Autodesk Fusion 360 part; units mm, degrees
(part 2 of 3)
sketch "Sketch2" plane through (0, 0, 0) normal (0, 0, -1) x (1, 0, 0)
  arc A0 (169.2125, 22.075) -> (169.7125, 21.575) centre (169.7125, 22.075) ccw
  line L0 (169.2125, 22.075) -> (169.2125, 35.075)
  arc A1 (169.7125, 35.575) -> (169.2125, 35.075) centre (169.7125, 35.075) ccw
  line L1 (169.7125, 35.575) -> (182.7125, 35.575)
  arc A2 (183.2125, 35.075) -> (182.7125, 35.575) centre (182.7125, 35.075) ccw
  line L2 (183.2125, 35.075) -> (183.2125, 22.075)
  arc A3 (182.7125, 21.575) -> (183.2125, 22.075) centre (182.7125, 22.075) ccw
  line L3 (182.7125, 21.575) -> (169.7125, 21.575)
  arc A4 (245.4125, 22.075) -> (245.9125, 21.575) centre (245.9125, 22.075) ccw
  line L4 (245.4125, 22.075) -> (245.4125, 35.075)
  arc A5 (245.9125, 35.575) -> (245.4125, 35.075) centre (245.9125, 35.075) ccw
  line L5 (245.9125, 35.575) -> (258.9125, 35.575)
  arc A6 (259.4125, 35.075) -> (258.9125, 35.575) centre (258.9125, 35.075) ccw
  line L6 (259.4125, 35.075) -> (259.4125, 22.075)
  arc A7 (258.9125, 21.575) -> (259.4125, 22.075) centre (258.9125, 22.075) ccw
  line L7 (258.9125, 21.575) -> (245.9125, 21.575)
  arc A8 (354.1625, 2.525) -> (354.6625, 3.025) centre (354.1625, 3.025) ccw
  line L8 (354.1625, 2.525) -> (341.1625, 2.525)
  arc A9 (340.6625, 3.025) -> (341.1625, 2.525) centre (341.1625, 3.025) ccw
  line L9 (340.6625, 3.025) -> (340.6625, 16.025)
  arc A10 (341.1625, 16.525) -> (340.6625, 16.025) centre (341.1625, 16.025) ccw
  line L10 (341.1625, 16.525) -> (354.1625, 16.525)
  arc A11 (354.6625, 16.025) -> (354.1625, 16.525) centre (354.1625, 16.025) ccw
  line L11 (354.6625, 16.025) -> (354.6625, 3.025)
  arc A12 (112.0625, 22.075) -> (112.5625, 21.575) centre (112.5625, 22.075) ccw
  line L12 (112.0625, 22.075) -> (112.0625, 35.075)
  arc A13 (112.5625, 35.575) -> (112.0625, 35.075) centre (112.5625, 35.075) ccw
  line L13 (112.5625, 35.575) -> (125.5625, 35.575)
  arc A14 (126.0625, 35.075) -> (125.5625, 35.575) centre (125.5625, 35.075) ccw
  line L14 (126.0625, 35.075) -> (126.0625, 22.075)
  arc A15 (125.5625, 21.575) -> (126.0625, 22.075) centre (125.5625, 22.075) ccw
  line L15 (125.5625, 21.575) -> (112.5625, 21.575)
  arc A16 (73.9625, 22.075) -> (74.4625, 21.575) centre (74.4625, 22.075) ccw
  line L16 (73.9625, 22.075) -> (73.9625, 35.075)
  arc A17 (74.4625, 35.575) -> (73.9625, 35.075) centre (74.4625, 35.075) ccw
  line L17 (74.4625, 35.575) -> (87.4625, 35.575)
  arc A18 (87.9625, 35.075) -> (87.4625, 35.575) centre (87.4625, 35.075) ccw
  line L18 (87.9625, 35.075) -> (87.9625, 22.075)
  arc A19 (87.4625, 21.575) -> (87.9625, 22.075) centre (87.4625, 22.075) ccw
  line L19 (87.4625, 21.575) -> (74.4625, 21.575)
  arc A20 (283.5125, 22.075) -> (284.0125, 21.575) centre (284.0125, 22.075) ccw
  line L20 (283.5125, 22.075) -> (283.5125, 35.075)
  arc A21 (284.0125, 35.575) -> (283.5125, 35.075) centre (284.0125, 35.075) ccw
  line L21 (284.0125, 35.575) -> (297.0125, 35.575)
  arc A22 (297.5125, 35.075) -> (297.0125, 35.575) centre (297.0125, 35.075) ccw
  line L22 (297.5125, 35.075) -> (297.5125, 22.075)
  arc A23 (297.0125, 21.575) -> (297.5125, 22.075) centre (297.0125, 22.075) ccw
  line L23 (297.0125, 21.575) -> (284.0125, 21.575)
  arc A24 (188.2625, 22.075) -> (188.7625, 21.575) centre (188.7625, 22.075) ccw
  line L24 (188.2625, 22.075) -> (188.2625, 35.075)
  arc A25 (188.7625, 35.575) -> (188.2625, 35.075) centre (188.7625, 35.075) ccw
  line L25 (188.7625, 35.575) -> (201.7625, 35.575)
  arc A26 (202.2625, 35.075) -> (201.7625, 35.575) centre (201.7625, 35.075) ccw
  line L26 (202.2625, 35.075) -> (202.2625, 22.075)
  arc A27 (201.7625, 21.575) -> (202.2625, 22.075) centre (201.7625, 22.075) ccw
  line L27 (201.7625, 21.575) -> (188.7625, 21.575)
  arc A28 (50.15, 22.075) -> (50.65, 21.575) centre (50.65, 22.075) ccw
  line L28 (50.15, 22.075) -> (50.15, 35.075)
  arc A29 (50.65, 35.575) -> (50.15, 35.075) centre (50.65, 35.075) ccw
  line L29 (50.65, 35.575) -> (63.65, 35.575)
  arc A30 (64.15, 35.075) -> (63.65, 35.575) centre (63.65, 35.075) ccw
  line L30 (64.15, 35.075) -> (64.15, 22.075)
  arc A31 (63.65, 21.575) -> (64.15, 22.075) centre (63.65, 22.075) ccw
  line L31 (63.65, 21.575) -> (50.65, 21.575)
  arc A32 (93.0125, 22.075) -> (93.5125, 21.575) centre (93.5125, 22.075) ccw
  line L32 (93.0125, 22.075) -> (93.0125, 35.075)
  arc A33 (93.5125, 35.575) -> (93.0125, 35.075) centre (93.5125, 35.075) ccw
  line L33 (93.5125, 35.575) -> (106.5125, 35.575)
  arc A34 (107.0125, 35.075) -> (106.5125, 35.575) centre (106.5125, 35.075) ccw
  line L34 (107.0125, 35.075) -> (107.0125, 22.075)
  arc A35 (106.5125, 21.575) -> (107.0125, 22.075) centre (106.5125, 22.075) ccw
  line L35 (106.5125, 21.575) -> (93.5125, 21.575)
  arc A36 (359.7125, 3.025) -> (360.2125, 2.525) centre (360.2125, 3.025) ccw
  line L36 (359.7125, 3.025) -> (359.7125, 16.025)
  arc A37 (360.2125, 16.525) -> (359.7125, 16.025) centre (360.2125, 16.025) ccw
  line L37 (360.2125, 16.525) -> (373.2125, 16.525)
  arc A38 (373.7125, 16.025) -> (373.2125, 16.525) centre (373.2125, 16.025) ccw
  line L38 (373.7125, 16.025) -> (373.7125, 3.025)
  arc A39 (373.2125, 2.525) -> (373.7125, 3.025) centre (373.2125, 3.025) ccw
  line L39 (373.2125, 2.525) -> (360.2125, 2.525)
  line L40 (131.1125, 22.075) -> (131.1125, 35.075)
  arc A40 (131.6125, 35.575) -> (131.1125, 35.075) centre (131.6125, 35.075) ccw
  line L41 (131.6125, 35.575) -> (144.6125, 35.575)
  arc A41 (145.1125, 35.075) -> (144.6125, 35.575) centre (144.6125, 35.075) ccw
  line L42 (145.1125, 35.075) -> (145.1125, 22.075)
  arc A42 (144.6125, 21.575) -> (145.1125, 22.075) centre (144.6125, 22.075) ccw
  line L43 (144.6125, 21.575) -> (131.6125, 21.575)
  arc A43 (131.1125, 22.075) -> (131.6125, 21.575) centre (131.6125, 22.075) ccw
  arc A44 (235.8875, 3.025) -> (236.3875, 2.525) centre (236.3875, 3.025) ccw
  line L44 (235.8875, 3.025) -> (235.8875, 16.025)
  arc A45 (236.3875, 16.525) -> (235.8875, 16.025) centre (236.3875, 16.025) ccw
  line L45 (236.3875, 16.525) -> (249.3875, 16.525)
  arc A46 (249.8875, 16.025) -> (249.3875, 16.525) centre (249.3875, 16.025) ccw
  line L46 (249.8875, 16.025) -> (249.8875, 3.025)
  arc A47 (249.3875, 2.525) -> (249.8875, 3.025) centre (249.3875, 3.025) ccw
  line L47 (249.3875, 2.525) -> (236.3875, 2.525)
  line L48 (207.3125, 22.075) -> (207.3125, 35.075)
  arc A48 (207.8125, 35.575) -> (207.3125, 35.075) centre (207.8125, 35.075) ccw
  line L49 (207.8125, 35.575) -> (220.8125, 35.575)
  arc A49 (221.3125, 35.075) -> (220.8125, 35.575) centre (220.8125, 35.075) ccw
  line L50 (221.3125, 35.075) -> (221.3125, 22.075)
  arc A50 (220.8125, 21.575) -> (221.3125, 22.075) centre (220.8125, 22.075) ccw
  line L51 (220.8125, 21.575) -> (207.8125, 21.575)
  arc A51 (207.3125, 22.075) -> (207.8125, 21.575) centre (207.8125, 22.075) ccw
  arc A52 (264.4625, 22.075) -> (264.9625, 21.575) centre (264.9625, 22.075) ccw
  line L52 (264.4625, 22.075) -> (264.4625, 35.075)
  arc A53 (264.9625, 35.575) -> (264.4625, 35.075) centre (264.9625, 35.075) ccw
  line L53 (264.9625, 35.575) -> (277.9625, 35.575)
  arc A54 (278.4625, 35.075) -> (277.9625, 35.575) centre (277.9625, 35.075) ccw
  line L54 (278.4625, 35.075) -> (278.4625, 22.075)
  arc A55 (277.9625, 21.575) -> (278.4625, 22.075) centre (277.9625, 22.075) ccw
  line L55 (277.9625, 21.575) -> (264.9625, 21.575)
  arc A56 (97.775, 41.125) -> (98.275, 40.625) centre (98.275, 41.125) ccw
  line L56 (97.775, 41.125) -> (97.775, 54.125)
  arc A57 (98.275, 54.625) -> (97.775, 54.125) centre (98.275, 54.125) ccw
  line L57 (98.275, 54.625) -> (111.275, 54.625)
  arc A58 (111.775, 54.125) -> (111.275, 54.625) centre (111.275, 54.125) ccw
  line L58 (111.775, 54.125) -> (111.775, 41.125)
  arc A59 (111.275, 40.625) -> (111.775, 41.125) centre (111.275, 41.125) ccw
  line L59 (111.275, 40.625) -> (98.275, 40.625)
  arc A60 (239.8625, 21.575) -> (240.3625, 22.075) centre (239.8625, 22.075) ccw
  line L60 (239.8625, 21.575) -> (226.8625, 21.575)
  arc A61 (226.3625, 22.075) -> (226.8625, 21.575) centre (226.8625, 22.075) ccw
  line L61 (226.3625, 22.075) -> (226.3625, 35.075)
  arc A62 (226.8625, 35.575) -> (226.3625, 35.075) centre (226.8625, 35.075) ccw
  line L62 (226.8625, 35.575) -> (239.8625, 35.575)
  arc A63 (240.3625, 35.075) -> (239.8625, 35.575) centre (239.8625, 35.075) ccw
  line L63 (240.3625, 35.075) -> (240.3625, 22.075)
  arc A64 (307.325, 22.075) -> (307.825, 21.575) centre (307.825, 22.075) ccw
  line L64 (307.325, 22.075) -> (307.325, 35.075)
  arc A65 (307.825, 35.575) -> (307.325, 35.075) centre (307.825, 35.075) ccw
  line L65 (307.825, 35.575) -> (320.825, 35.575)
  arc A66 (321.325, 35.075) -> (320.825, 35.575) centre (320.825, 35.075) ccw
  line L66 (321.325, 35.075) -> (321.325, 22.075)
  arc A67 (320.825, 21.575) -> (321.325, 22.075) centre (320.825, 22.075) ccw
  line L67 (320.825, 21.575) -> (307.825, 21.575)
  arc A68 (116.825, 41.125) -> (117.325, 40.625) centre (117.325, 41.125) ccw
  line L68 (116.825, 41.125) -> (116.825, 54.125)
  arc A69 (117.325, 54.625) -> (116.825, 54.125) centre (117.325, 54.125) ccw
  line L69 (117.325, 54.625) -> (130.325, 54.625)
  arc A70 (130.825, 54.125) -> (130.325, 54.625) centre (130.325, 54.125) ccw
  line L70 (130.825, 54.125) -> (130.825, 41.125)
  arc A71 (130.325, 40.625) -> (130.825, 41.125) centre (130.325, 41.125) ccw
  line L71 (130.325, 40.625) -> (117.325, 40.625)
  arc A72 (354.1625, 21.575) -> (354.6625, 22.075) centre (354.1625, 22.075) ccw
  line L72 (354.1625, 21.575) -> (341.1625, 21.575)
  arc A73 (340.6625, 22.075) -> (341.1625, 21.575) centre (341.1625, 22.075) ccw
  line L73 (340.6625, 22.075) -> (340.6625, 35.075)
  arc A74 (341.1625, 35.575) -> (340.6625, 35.075) centre (341.1625, 35.075) ccw
  line L74 (341.1625, 35.575) -> (354.1625, 35.575)
  arc A75 (354.6625, 35.075) -> (354.1625, 35.575) centre (354.1625, 35.075) ccw
  line L75 (354.6625, 35.075) -> (354.6625, 22.075)
  arc A76 (359.7125, 22.075) -> (360.2125, 21.575) centre (360.2125, 22.075) ccw
  line L76 (359.7125, 22.075) -> (359.7125, 35.075)
  arc A77 (360.2125, 35.575) -> (359.7125, 35.075) centre (360.2125, 35.075) ccw
  line L77 (360.2125, 35.575) -> (373.2125, 35.575)
  arc A78 (373.7125, 35.075) -> (373.2125, 35.575) centre (373.2125, 35.075) ccw
  line L78 (373.7125, 35.075) -> (373.7125, 22.075)
  arc A79 (373.2125, 21.575) -> (373.7125, 22.075) centre (373.2125, 22.075) ccw
  line L79 (373.2125, 21.575) -> (360.2125, 21.575)
  arc A80 (163.6625, 21.575) -> (164.1625, 22.075) centre (163.6625, 22.075) ccw
  line L80 (163.6625, 21.575) -> (150.6625, 21.575)
  arc A81 (150.1625, 22.075) -> (150.6625, 21.575) centre (150.6625, 22.075) ccw
  line L81 (150.1625, 22.075) -> (150.1625, 35.075)
  arc A82 (150.6625, 35.575) -> (150.1625, 35.075) centre (150.6625, 35.075) ccw
  line L82 (150.6625, 35.575) -> (163.6625, 35.575)
  arc A83 (164.1625, 35.075) -> (163.6625, 35.575) centre (163.6625, 35.075) ccw
  line L83 (164.1625, 35.075) -> (164.1625, 22.075)
  arc A84 (92.225, 40.625) -> (92.725, 41.125) centre (92.225, 41.125) ccw
  line L84 (92.225, 40.625) -> (79.225, 40.625)
  arc A85 (78.725, 41.125) -> (79.225, 40.625) centre (79.225, 41.125) ccw
  line L85 (78.725, 41.125) -> (78.725, 54.125)
  arc A86 (79.225, 54.625) -> (78.725, 54.125) centre (79.225, 54.125) ccw
  line L86 (79.225, 54.625) -> (92.225, 54.625)
  arc A87 (92.725, 54.125) -> (92.225, 54.625) centre (92.225, 54.125) ccw
  line L87 (92.725, 54.125) -> (92.725, 41.125)
  line L88 (45.3875, 41.125) -> (45.3875, 54.125)
  arc A88 (45.8875, 54.625) -> (45.3875, 54.125) centre (45.8875, 54.125) ccw
  line L89 (45.8875, 54.625) -> (66.0312, 54.625)
  arc A89 (66.5312, 54.125) -> (66.0312, 54.625) centre (66.0312, 54.125) ccw
  line L90 (66.5312, 54.125) -> (66.5312, 41.125)
  arc A90 (66.0312, 40.625) -> (66.5312, 41.125) centre (66.0312, 41.125) ccw
  line L91 (66.0312, 40.625) -> (45.8875, 40.625)
  arc A91 (45.3875, 41.125) -> (45.8875, 40.625) centre (45.8875, 41.125) ccw
  arc A92 (121.5875, 3.025) -> (122.0875, 2.525) centre (122.0875, 3.025) ccw
  line L92 (121.5875, 3.025) -> (121.5875, 16.025)
  arc A93 (122.0875, 16.525) -> (121.5875, 16.025) centre (122.0875, 16.025) ccw
  line L93 (122.0875, 16.525) -> (135.0875, 16.525)
  arc A94 (135.5875, 16.025) -> (135.0875, 16.525) centre (135.0875, 16.025) ccw
  line L94 (135.5875, 16.025) -> (135.5875, 3.025)
  arc A95 (135.0875, 2.525) -> (135.5875, 3.025) centre (135.0875, 3.025) ccw
  line L95 (135.0875, 2.525) -> (122.0875, 2.525)
  arc A96 (250.175, 41.125) -> (250.675, 40.625) centre (250.675, 41.125) ccw
  line L96 (250.175, 41.125) -> (250.175, 54.125)
  arc A97 (250.675, 54.625) -> (250.175, 54.125) centre (250.675, 54.125) ccw
  line L97 (250.675, 54.625) -> (263.675, 54.625)
  arc A98 (264.175, 54.125) -> (263.675, 54.625) centre (263.675, 54.125) ccw
  line L98 (264.175, 54.125) -> (264.175, 41.125)
  arc A99 (263.675, 40.625) -> (264.175, 41.125) centre (263.675, 41.125) ccw
  line L99 (263.675, 40.625) -> (250.675, 40.625)
  arc A100 (187.475, 40.625) -> (187.975, 41.125) centre (187.475, 41.125) ccw
  line L100 (187.475, 40.625) -> (174.475, 40.625)
  arc A101 (173.975, 41.125) -> (174.475, 40.625) centre (174.475, 41.125) ccw
  line L101 (173.975, 41.125) -> (173.975, 54.125)
  arc A102 (174.475, 54.625) -> (173.975, 54.125) centre (174.475, 54.125) ccw
  line L102 (174.475, 54.625) -> (187.475, 54.625)
  arc A103 (187.975, 54.125) -> (187.475, 54.625) centre (187.475, 54.125) ccw
  line L103 (187.975, 54.125) -> (187.975, 41.125)
  arc A104 (154.925, 41.125) -> (155.425, 40.625) centre (155.425, 41.125) ccw
  line L104 (154.925, 41.125) -> (154.925, 54.125)
  arc A105 (155.425, 54.625) -> (154.925, 54.125) centre (155.425, 54.125) ccw
  line L105 (155.425, 54.625) -> (168.425, 54.625)
  arc A106 (168.925, 54.125) -> (168.425, 54.625) centre (168.425, 54.125) ccw
  line L106 (168.925, 54.125) -> (168.925, 41.125)
  arc A107 (168.425, 40.625) -> (168.925, 41.125) centre (168.425, 41.125) ccw
  line L107 (168.425, 40.625) -> (155.425, 40.625)
  arc A108 (315.6193, 42.125) -> (316.1193, 41.625) centre (316.1193, 42.125) ccw
  line L108 (315.6193, 42.125) -> (315.6193, 56.125)
  arc A109 (316.1193, 56.625) -> (315.6193, 56.125) centre (316.1193, 56.125) ccw
  line L109 (316.1193, 56.625) -> (322.1193, 56.625)
  arc A110 (322.6192, 56.125) -> (322.1193, 56.625) centre (322.1193, 56.125) ccw
  line L110 (322.6192, 56.125) -> (322.6192, 42.125)
  arc A111 (322.1193, 41.625) -> (322.6192, 42.125) centre (322.1193, 42.125) ccw
  line L111 (322.1193, 41.625) -> (316.1193, 41.625)
  arc A112 (72.7318, 61.175) -> (73.2318, 60.675) centre (73.2318, 61.175) ccw
  line L112 (72.7318, 61.175) -> (72.7318, 75.175)
  arc A113 (73.2318, 75.675) -> (72.7318, 75.175) centre (73.2318, 75.175) ccw
  line L113 (73.2318, 75.675) -> (79.2318, 75.675)
  arc A114 (79.7318, 75.175) -> (79.2318, 75.675) centre (79.2318, 75.175) ccw
  line L114 (79.7318, 75.175) -> (79.7318, 61.175)
  arc A115 (79.2318, 60.675) -> (79.7318, 61.175) centre (79.2318, 61.175) ccw
  line L115 (79.2318, 60.675) -> (73.2318, 60.675)
  arc A116 (139.85, 59.675) -> (140.35, 60.175) centre (139.85, 60.175) ccw
  line L116 (139.85, 59.675) -> (126.85, 59.675)
  arc A117 (126.35, 60.175) -> (126.85, 59.675) centre (126.85, 60.175) ccw
  line L117 (126.35, 60.175) -> (126.35, 73.175)
  arc A118 (126.85, 73.675) -> (126.35, 73.175) centre (126.85, 73.175) ccw
  line L118 (126.85, 73.675) -> (139.85, 73.675)
  arc A119 (140.35, 73.175) -> (139.85, 73.675) centre (139.85, 73.175) ccw
  line L119 (140.35, 73.175) -> (140.35, 60.175)
  line L120 (145.4, 60.175) -> (145.4, 73.175)
  arc A120 (145.9, 73.675) -> (145.4, 73.175) centre (145.9, 73.175) ccw
  line L121 (145.9, 73.675) -> (158.9, 73.675)
  arc A121 (159.4, 73.175) -> (158.9, 73.675) centre (158.9, 73.175) ccw
  line L122 (159.4, 73.175) -> (159.4, 60.175)
  arc A122 (158.9, 59.675) -> (159.4, 60.175) centre (158.9, 60.175) ccw
  line L123 (158.9, 59.675) -> (145.9, 59.675)
  arc A123 (145.4, 60.175) -> (145.9, 59.675) centre (145.9, 60.175) ccw
  arc A124 (183.5, 60.175) -> (184, 59.675) centre (184, 60.175) ccw
  line L124 (183.5, 60.175) -> (183.5, 73.175)
  arc A125 (184, 73.675) -> (183.5, 73.175) centre (184, 73.175) ccw
  line L125 (184, 73.675) -> (197, 73.675)
  arc A126 (197.5, 73.175) -> (197, 73.675) centre (197, 73.175) ccw
  line L126 (197.5, 73.175) -> (197.5, 60.175)
  arc A127 (197, 59.675) -> (197.5, 60.175) centre (197, 60.175) ccw
  line L127 (197, 59.675) -> (184, 59.675)
  arc A128 (48.8558, 61.175) -> (49.3558, 60.675) centre (49.3558, 61.175) ccw
  line L128 (48.8558, 61.175) -> (48.8558, 75.175)
  arc A129 (49.3558, 75.675) -> (48.8558, 75.175) centre (49.3558, 75.175) ccw
  line L129 (49.3558, 75.675) -> (55.3558, 75.675)
  arc A130 (55.8558, 75.175) -> (55.3558, 75.675) centre (55.3558, 75.175) ccw
  line L130 (55.8558, 75.175) -> (55.8558, 61.175)
  arc A131 (55.3558, 60.675) -> (55.8558, 61.175) centre (55.3558, 61.175) ccw
  line L131 (55.3558, 60.675) -> (49.3558, 60.675)
  arc A132 (340.6625, 60.175) -> (341.1625, 59.675) centre (341.1625, 60.175) ccw
  line L132 (340.6625, 60.175) -> (340.6625, 73.175)
  arc A133 (341.1625, 73.675) -> (340.6625, 73.175) centre (341.1625, 73.175) ccw
  line L133 (341.1625, 73.675) -> (354.1625, 73.675)
  arc A134 (354.6625, 73.175) -> (354.1625, 73.675) centre (354.1625, 73.175) ccw
  line L134 (354.6625, 73.175) -> (354.6625, 60.175)
  arc A135 (354.1625, 59.675) -> (354.6625, 60.175) centre (354.1625, 60.175) ccw
  line L135 (354.1625, 59.675) -> (341.1625, 59.675)
  arc A136 (164.45, 60.175) -> (164.95, 59.675) centre (164.95, 60.175) ccw
  line L136 (164.45, 60.175) -> (164.45, 73.175)
  arc A137 (164.95, 73.675) -> (164.45, 73.175) centre (164.95, 73.175) ccw
  line L137 (164.95, 73.675) -> (177.95, 73.675)
  arc A138 (178.45, 73.175) -> (177.95, 73.675) centre (177.95, 73.175) ccw
  line L138 (178.45, 73.175) -> (178.45, 60.175)
  arc A139 (177.95, 59.675) -> (178.45, 60.175) centre (177.95, 60.175) ccw
  line L139 (177.95, 59.675) -> (164.95, 59.675)
  arc A140 (259.7, 60.175) -> (260.2, 59.675) centre (260.2, 60.175) ccw
  line L140 (259.7, 60.175) -> (259.7, 73.175)
  arc A141 (260.2, 73.675) -> (259.7, 73.175) centre (260.2, 73.175) ccw
  line L141 (260.2, 73.675) -> (273.2, 73.675)
  arc A142 (273.7, 73.175) -> (273.2, 73.675) centre (273.2, 73.175) ccw
  line L142 (273.7, 73.175) -> (273.7, 60.175)
  arc A143 (273.2, 59.675) -> (273.7, 60.175) centre (273.2, 60.175) ccw
  line L143 (273.2, 59.675) -> (260.2, 59.675)
  arc A144 (313.6812, 40.625) -> (314.1812, 41.125) centre (313.6812, 41.125) ccw
  line L144 (313.6812, 40.625) -> (300.6812, 40.625)
  arc A145 (300.1812, 41.125) -> (300.6812, 40.625) centre (300.6812, 41.125) ccw
  line L145 (300.1812, 41.125) -> (300.1812, 54.125)
  arc A146 (300.6812, 54.625) -> (300.1812, 54.125) centre (300.6812, 54.125) ccw
  line L146 (300.6812, 54.625) -> (313.6812, 54.625)
  arc A147 (314.1812, 54.125) -> (313.6812, 54.625) centre (313.6812, 54.125) ccw
  line L147 (314.1812, 54.125) -> (314.1812, 41.125)
  arc A148 (135.875, 41.125) -> (136.375, 40.625) centre (136.375, 41.125) ccw
  line L148 (135.875, 41.125) -> (135.875, 54.125)
  arc A149 (136.375, 54.625) -> (135.875, 54.125) centre (136.375, 54.125) ccw
  line L149 (136.375, 54.625) -> (149.375, 54.625)
  arc A150 (149.875, 54.125) -> (149.375, 54.625) centre (149.375, 54.125) ccw
  line L150 (149.875, 54.125) -> (149.875, 41.125)
  arc A151 (149.375, 40.625) -> (149.875, 41.125) centre (149.375, 41.125) ccw
  line L151 (149.375, 40.625) -> (136.375, 40.625)
  arc A152 (166.8313, 79.225) -> (167.3313, 78.725) centre (167.3313, 79.225) ccw
  line L152 (166.8313, 79.225) -> (166.8313, 92.225)
  arc A153 (167.3313, 92.725) -> (166.8313, 92.225) centre (167.3313, 92.225) ccw
  line L153 (167.3313, 92.725) -> (180.3313, 92.725)
  arc A154 (180.8313, 92.225) -> (180.3313, 92.725) centre (180.3313, 92.225) ccw
  line L154 (180.8313, 92.225) -> (180.8313, 79.225)
  arc A155 (180.3313, 78.725) -> (180.8313, 79.225) centre (180.3313, 79.225) ccw
  line L155 (180.3313, 78.725) -> (167.3313, 78.725)
  line L156 (107.3, 60.175) -> (107.3, 73.175)
  arc A156 (107.8, 73.675) -> (107.3, 73.175) centre (107.8, 73.175) ccw
  line L157 (107.8, 73.675) -> (120.8, 73.675)
  arc A157 (121.3, 73.175) -> (120.8, 73.675) centre (120.8, 73.175) ccw
  line L158 (121.3, 73.175) -> (121.3, 60.175)
  arc A158 (120.8, 59.675) -> (121.3, 60.175) centre (120.8, 60.175) ccw
  line L159 (120.8, 59.675) -> (107.8, 59.675)
  arc A159 (107.3, 60.175) -> (107.8, 59.675) centre (107.8, 60.175) ccw
  arc A160 (291.7432, 42.125) -> (292.2432, 41.625) centre (292.2432, 42.125) ccw
  line L160 (291.7432, 42.125) -> (291.7432, 56.125)
  arc A161 (292.2432, 56.625) -> (291.7432, 56.125) centre (292.2432, 56.125) ccw
  line L161 (292.2432, 56.625) -> (298.2432, 56.625)
  arc A162 (298.7432, 56.125) -> (298.2432, 56.625) centre (298.2432, 56.125) ccw
  line L162 (298.7433, 56.125) -> (298.7433, 42.125)
  arc A163 (298.2432, 41.625) -> (298.7432, 42.125) centre (298.2432, 42.125) ccw
  line L163 (298.2432, 41.625) -> (292.2432, 41.625)
  arc A164 (220.3313, 80.225) -> (220.8313, 79.725) centre (220.8313, 80.225) ccw
  line L164 (220.3313, 80.225) -> (220.3313, 94.225)
  arc A165 (220.8313, 94.725) -> (220.3313, 94.225) centre (220.8313, 94.225) ccw
  line L165 (220.8313, 94.725) -> (226.8313, 94.725)
  arc A166 (227.3313, 94.225) -> (226.8313, 94.725) centre (226.8313, 94.225) ccw
  line L166 (227.3313, 94.225) -> (227.3313, 80.225)
  arc A167 (226.8313, 79.725) -> (227.3313, 80.225) centre (226.8313, 80.225) ccw
  line L167 (226.8313, 79.725) -> (220.8313, 79.725)
  arc A168 (120.3313, 80.225) -> (120.8313, 79.725) centre (120.8313, 80.225) ccw
  line L168 (120.3313, 80.225) -> (120.3312, 94.225)
  arc A169 (120.8313, 94.725) -> (120.3313, 94.225) centre (120.8313, 94.225) ccw
  line L169 (120.8313, 94.725) -> (126.8313, 94.725)
  arc A170 (127.3313, 94.225) -> (126.8313, 94.725) centre (126.8313, 94.225) ccw
  line L170 (127.3313, 94.225) -> (127.3313, 80.225)
  arc A171 (126.8313, 79.725) -> (127.3313, 80.225) centre (126.8313, 80.225) ccw
  line L171 (126.8313, 79.725) -> (120.8313, 79.725)
  arc A172 (95.3938, 79.225) -> (95.8938, 78.725) centre (95.8938, 79.225) ccw
  line L172 (95.3937, 79.225) -> (95.3937, 92.225)
  arc A173 (95.8938, 92.725) -> (95.3938, 92.225) centre (95.8938, 92.225) ccw
  line L173 (95.8938, 92.725) -> (108.8938, 92.725)
  arc A174 (109.3938, 92.225) -> (108.8938, 92.725) centre (108.8938, 92.225) ccw
  line L174 (109.3938, 92.225) -> (109.3938, 79.225)
  arc A175 (108.8938, 78.725) -> (109.3938, 79.225) centre (108.8938, 79.225) ccw
  line L175 (108.8938, 78.725) -> (95.8938, 78.725)
  arc A176 (202.55, 60.175) -> (203.05, 59.675) centre (203.05, 60.175) ccw
  line L176 (202.55, 60.175) -> (202.55, 73.175)
  arc A177 (203.05, 73.675) -> (202.55, 73.175) centre (203.05, 73.175) ccw
  line L177 (203.05, 73.675) -> (216.05, 73.675)
  arc A178 (216.55, 73.175) -> (216.05, 73.675) centre (216.05, 73.175) ccw
  line L178 (216.55, 73.175) -> (216.55, 60.175)
  arc A179 (216.05, 59.675) -> (216.55, 60.175) centre (216.05, 60.175) ccw
  line L179 (216.05, 59.675) -> (203.05, 59.675)
  arc A180 (88.25, 60.175) -> (88.75, 59.675) centre (88.75, 60.175) ccw
  line L180 (88.25, 60.175) -> (88.25, 73.175)
  arc A181 (88.75, 73.675) -> (88.25, 73.175) centre (88.75, 73.175) ccw
  line L181 (88.75, 73.675) -> (101.75, 73.675)
  arc A182 (102.25, 73.175) -> (101.75, 73.675) centre (101.75, 73.175) ccw
  line L182 (102.25, 73.175) -> (102.25, 60.175)
  arc A183 (101.75, 59.675) -> (102.25, 60.175) centre (101.75, 60.175) ccw
  line L183 (101.75, 59.675) -> (88.75, 59.675)
  line L184 (240.65, 60.175) -> (240.65, 73.175)
  arc A184 (241.15, 73.675) -> (240.65, 73.175) centre (241.15, 73.175) ccw
  line L185 (241.15, 73.675) -> (254.15, 73.675)
  arc A185 (254.65, 73.175) -> (254.15, 73.675) centre (254.15, 73.175) ccw
  line L186 (254.65, 73.175) -> (254.65, 60.175)
  arc A186 (254.15, 59.675) -> (254.65, 60.175) centre (254.15, 60.175) ccw
  line L187 (254.15, 59.675) -> (241.15, 59.675)
  arc A187 (240.65, 60.175) -> (241.15, 59.675) centre (241.15, 60.175) ccw
  arc A188 (221.6, 60.175) -> (222.1, 59.675) centre (222.1, 60.175) ccw
  line L188 (221.6, 60.175) -> (221.6, 73.175)
  arc A189 (222.1, 73.675) -> (221.6, 73.175) centre (222.1, 73.175) ccw
  line L189 (222.1, 73.675) -> (235.1, 73.675)
  arc A190 (235.6, 73.175) -> (235.1, 73.675) centre (235.1, 73.175) ccw
  line L190 (235.6, 73.175) -> (235.6, 60.175)
  arc A191 (235.1, 59.675) -> (235.6, 60.175) centre (235.1, 60.175) ccw
  line L191 (235.1, 59.675) -> (222.1, 59.675)
  arc A192 (262.0813, 79.225) -> (262.5813, 78.725) centre (262.5813, 79.225) ccw
  line L192 (262.0813, 79.225) -> (262.0813, 92.225)
  arc A193 (262.5813, 92.725) -> (262.0813, 92.225) centre (262.5813, 92.225) ccw
  line L193 (262.5813, 92.725) -> (275.5813, 92.725)
  arc A194 (276.0813, 92.225) -> (275.5813, 92.725) centre (275.5813, 92.225) ccw
  line L194 (276.0813, 92.225) -> (276.0813, 79.225)
  arc A195 (275.5813, 78.725) -> (276.0813, 79.225) centre (275.5813, 79.225) ccw
  line L195 (275.5813, 78.725) -> (262.5813, 78.725)
  arc A196 (231.125, 41.125) -> (231.625, 40.625) centre (231.625, 41.125) ccw
  line L196 (231.125, 41.125) -> (231.125, 54.125)
  arc A197 (231.625, 54.625) -> (231.125, 54.125) centre (231.625, 54.125) ccw
  line L197 (231.625, 54.625) -> (244.625, 54.625)
  arc A198 (245.125, 54.125) -> (244.625, 54.625) centre (244.625, 54.125) ccw
  line L198 (245.125, 54.125) -> (245.125, 41.125)
  arc A199 (244.625, 40.625) -> (245.125, 41.125) centre (244.625, 41.125) ccw
  line L199 (244.625, 40.625) -> (231.625, 40.625)
  arc A200 (71.5812, 79.225) -> (72.0812, 78.725) centre (72.0812, 79.225) ccw
  line L200 (71.5812, 79.225) -> (71.5812, 92.225)
  arc A201 (72.0812, 92.725) -> (71.5812, 92.225) centre (72.0812, 92.225) ccw
  line L201 (72.0812, 92.725) -> (85.0812, 92.725)
  arc A202 (85.5813, 92.225) -> (85.0812, 92.725) centre (85.0812, 92.225) ccw
  line L202 (85.5813, 92.225) -> (85.5813, 79.225)
  arc A203 (85.0812, 78.725) -> (85.5813, 79.225) centre (85.0812, 79.225) ccw
  line L203 (85.0812, 78.725) -> (72.0812, 78.725)
  arc A204 (463.5139, 44.7152) -> (463.5139, 48.8568) centre (463.5139, 46.786) ccw
  line L204 (463.5139, 44.7152) -> (459.7929, 44.7152)
  line L205 (459.7929, 44.7152) -> (459.7929, 34.7152)
  line L206 (459.7929, 34.7152) -> (383.7929, 34.7152)
  line L207 (383.7929, 34.7152) -> (383.7929, 44.7152)
  line L208 (383.7929, 44.7152) -> (380.072, 44.7152)
  arc A205 (380.072, 48.8568) -> (380.072, 44.7152) centre (380.072, 46.786) ccw
  line L209 (380.072, 48.8568) -> (383.7929, 48.8568)
  line L210 (383.7929, 48.8568) -> (383.7929, 88.7152)
  line L211 (383.7929, 88.7152) -> (459.7929, 88.7152)
  line L212 (459.7929, 88.7152) -> (459.7929, 48.8568)
  line L213 (459.7929, 48.8568) -> (463.5139, 48.8568)
  arc A206 (287.4808, 75.675) -> (286.9808, 75.175) centre (287.4808, 75.175) ccw
  line L214 (287.4808, 75.675) -> (293.4808, 75.675)
  arc A207 (293.9808, 75.175) -> (293.4808, 75.675) centre (293.4808, 75.175) ccw
  line L215 (293.9808, 75.175) -> (293.9808, 74.175)
  arc A208 (293.9808, 74.175) -> (294.4808, 73.675) centre (294.4807, 74.175) ccw
  line L216 (294.4808, 73.675) -> (308.9188, 73.675)
  arc A209 (309.4187, 73.175) -> (308.9187, 73.675) centre (308.9187, 73.175) ccw
  line L217 (309.4187, 73.175) -> (309.4187, 60.175)
  arc A210 (308.9187, 59.675) -> (309.4187, 60.175) centre (308.9187, 60.175) ccw
  line L218 (308.9187, 59.675) -> (286.3937, 59.675)
  arc A211 (285.8937, 60.175) -> (286.3937, 59.675) centre (286.3937, 60.175) ccw
  line L219 (285.8937, 60.175) -> (285.8938, 73.175)
  arc A212 (286.3937, 73.675) -> (285.8937, 73.175) centre (286.3937, 73.175) ccw
  line L220 (286.3937, 73.675) -> (286.4808, 73.675)
  arc A213 (286.4808, 73.675) -> (286.9808, 74.175) centre (286.4808, 74.175) ccw
  line L221 (286.9808, 74.175) -> (286.9808, 75.175)
  arc A214 (238.2688, 79.225) -> (238.7688, 78.725) centre (238.7688, 79.225) ccw
  line L222 (238.2688, 79.225) -> (238.2688, 92.225)
  arc A215 (238.7688, 92.725) -> (238.2688, 92.225) centre (238.7688, 92.225) ccw
  line L223 (238.7688, 92.725) -> (251.7687, 92.725)
  arc A216 (252.2687, 92.225) -> (251.7687, 92.725) centre (251.7687, 92.225) ccw
  line L224 (252.2688, 92.225) -> (252.2688, 79.225)
  arc A217 (251.7687, 78.725) -> (252.2687, 79.225) centre (251.7687, 79.225) ccw
  line L225 (251.7687, 78.725) -> (238.7688, 78.725)
  line L226 (273.9875, 3.025) -> (273.9875, 16.025)
  arc A218 (274.4875, 16.525) -> (273.9875, 16.025) centre (274.4875, 16.025) ccw
  line L227 (274.4875, 16.525) -> (287.4875, 16.525)
  arc A219 (287.9875, 16.025) -> (287.4875, 16.525) centre (287.4875, 16.025) ccw
  line L228 (287.9875, 16.025) -> (287.9875, 3.025)
  arc A220 (287.4875, 2.525) -> (287.9875, 3.025) centre (287.4875, 3.025) ccw
  line L229 (287.4875, 2.525) -> (274.4875, 2.525)
  arc A221 (273.9875, 3.025) -> (274.4875, 2.525) centre (274.4875, 3.025) ccw
  arc A222 (326.0875, 73.175) -> (325.5875, 73.675) centre (325.5875, 73.175) ccw
  line L230 (326.0875, 73.175) -> (326.0875, 60.175)
  arc A223 (325.5875, 59.675) -> (326.0875, 60.175) centre (325.5875, 60.175) ccw
  line L231 (325.5875, 59.675) -> (312.5875, 59.675)
  arc A224 (312.0875, 60.175) -> (312.5875, 59.675) centre (312.5875, 60.175) ccw
  arc A225 (312.0875, 60.175) -> (311.5875, 60.675) centre (311.5875, 60.175) ccw
  line L232 (311.5875, 60.675) -> (311.3567, 60.675)
  arc A226 (310.8567, 61.175) -> (311.3567, 60.675) centre (311.3567, 61.175) ccw
  line L233 (310.8567, 61.175) -> (310.8567, 75.175)
  arc A227 (311.3567, 75.675) -> (310.8567, 75.175) centre (311.3567, 75.175) ccw
  line L234 (311.3567, 75.675) -> (317.3567, 75.675)
  arc A228 (317.8568, 75.175) -> (317.3568, 75.675) centre (317.3568, 75.175) ccw
  line L235 (317.8568, 75.175) -> (317.8568, 74.175)
  arc A229 (317.8568, 74.175) -> (318.3568, 73.675) centre (318.3567, 74.175) ccw
  line L236 (318.3568, 73.675) -> (325.5875, 73.675)
  arc A230 (254.9375, 3.025) -> (255.4375, 2.525) centre (255.4375, 3.025) ccw
  line L237 (254.9375, 3.025) -> (254.9375, 16.025)
  arc A231 (255.4375, 16.525) -> (254.9375, 16.025) centre (255.4375, 16.025) ccw
  line L238 (255.4375, 16.525) -> (268.4375, 16.525)
  arc A232 (268.9375, 16.025) -> (268.4375, 16.525) centre (268.4375, 16.025) ccw
  line L239 (268.9375, 16.025) -> (268.9375, 3.025)
  arc A233 (268.4375, 2.525) -> (268.9375, 3.025) centre (268.4375, 3.025) ccw
  line L240 (268.4375, 2.525) -> (255.4375, 2.525)
  arc A234 (326.0875, 16.025) -> (325.5875, 16.525) centre (325.5875, 16.025) ccw
  line L241 (326.0875, 16.025) -> (326.0875, 3.025)
  arc A235 (325.5875, 2.525) -> (326.0875, 3.025) centre (325.5875, 3.025) ccw
  line L242 (325.5875, 2.525) -> (293.5375, 2.525)
  arc A236 (293.0375, 3.025) -> (293.5375, 2.525) centre (293.5375, 3.025) ccw
  line L243 (293.0375, 3.025) -> (293.0375, 16.025)
  arc A237 (293.5375, 16.525) -> (293.0375, 16.025) centre (293.5375, 16.025) ccw
  line L244 (293.5375, 16.525) -> (293.6245, 16.525)
  arc A238 (293.6245, 16.525) -> (294.1245, 17.025) centre (293.6245, 17.025) ccw
  line L245 (294.1245, 17.025) -> (294.1245, 18.025)
  arc A239 (294.6245, 18.525) -> (294.1245, 18.025) centre (294.6245, 18.025) ccw
  line L246 (294.6245, 18.525) -> (300.6245, 18.525)
  arc A240 (301.1245, 18.025) -> (300.6245, 18.525) centre (300.6245, 18.025) ccw
  line L247 (301.1245, 18.025) -> (301.1245, 17.025)
  arc A241 (301.1245, 17.025) -> (301.6245, 16.525) centre (301.6245, 17.025) ccw
  line L248 (301.6245, 16.525) -> (317.5005, 16.525)
  arc A242 (317.5005, 16.525) -> (318.0005, 17.025) centre (317.5005, 17.025) ccw
  line L249 (318.0005, 17.025) -> (318.0005, 18.025)
  arc A243 (318.5005, 18.525) -> (318.0005, 18.025) centre (318.5005, 18.025) ccw
  line L250 (318.5005, 18.525) -> (324.5005, 18.525)
  arc A244 (325.0005, 18.025) -> (324.5005, 18.525) centre (324.5005, 18.025) ccw
  line L251 (325.0005, 18.025) -> (325.0005, 17.025)
  arc A245 (325.0005, 17.025) -> (325.5005, 16.525) centre (325.5005, 17.025) ccw
  line L252 (325.5005, 16.525) -> (325.5875, 16.525)
  arc A246 (212.075, 41.125) -> (212.575, 40.625) centre (212.575, 41.125) ccw
  line L253 (212.075, 41.125) -> (212.075, 54.125)
  arc A247 (212.575, 54.625) -> (212.075, 54.125) centre (212.575, 54.125) ccw
  line L254 (212.575, 54.625) -> (225.575, 54.625)
  arc A248 (226.075, 54.125) -> (225.575, 54.625) centre (225.575, 54.125) ccw
  line L255 (226.075, 54.125) -> (226.075, 41.125)
  arc A249 (225.575, 40.625) -> (226.075, 41.125) centre (225.575, 41.125) ccw
  line L256 (225.575, 40.625) -> (212.575, 40.625)
  arc A250 (57.2938, 60.175) -> (57.7938, 59.675) centre (57.7938, 60.175) ccw
  line L257 (57.2938, 60.175) -> (57.2938, 73.175)
  arc A251 (57.7938, 73.675) -> (57.2938, 73.175) centre (57.7938, 73.175) ccw
  line L258 (57.7938, 73.675) -> (70.7938, 73.675)
  arc A252 (71.2938, 73.175) -> (70.7938, 73.675) centre (70.7938, 73.175) ccw
  line L259 (71.2938, 73.175) -> (71.2938, 60.175)
  arc A253 (70.7938, 59.675) -> (71.2938, 60.175) centre (70.7938, 60.175) ccw
  line L260 (70.7938, 59.675) -> (57.7938, 59.675)
  arc A254 (321.6125, 79.225) -> (322.1125, 78.725) centre (322.1125, 79.225) ccw
  line L261 (321.6125, 79.225) -> (321.6125, 92.225)
  arc A255 (322.1125, 92.725) -> (321.6125, 92.225) centre (322.1125, 92.225) ccw
  line L262 (322.1125, 92.725) -> (335.1125, 92.725)
  arc A256 (335.6125, 92.225) -> (335.1125, 92.725) centre (335.1125, 92.225) ccw
  line L263 (335.6125, 92.225) -> (335.6125, 79.225)
  arc A257 (335.1125, 78.725) -> (335.6125, 79.225) centre (335.1125, 79.225) ccw
  line L264 (335.1125, 78.725) -> (322.1125, 78.725)
  arc A258 (193.025, 41.125) -> (193.525, 40.625) centre (193.525, 41.125) ccw
  line L265 (193.025, 41.125) -> (193.025, 54.125)
  arc A259 (193.525, 54.625) -> (193.025, 54.125) centre (193.525, 54.125) ccw
  line L266 (193.525, 54.625) -> (206.525, 54.625)
  arc A260 (207.025, 54.125) -> (206.525, 54.625) centre (206.525, 54.125) ccw
  line L267 (207.025, 54.125) -> (207.025, 41.125)
  arc A261 (206.525, 40.625) -> (207.025, 41.125) centre (206.525, 41.125) ccw
  line L268 (206.525, 40.625) -> (193.525, 40.625)
  arc A262 (285.8938, 79.225) -> (286.3938, 78.725) centre (286.3938, 79.225) ccw
  line L269 (285.8938, 79.225) -> (285.8938, 92.225)
  arc A263 (286.3938, 92.725) -> (285.8938, 92.225) centre (286.3938, 92.225) ccw
  line L270 (286.3938, 92.725) -> (299.3938, 92.725)
  arc A264 (299.8938, 92.225) -> (299.3938, 92.725) centre (299.3938, 92.225) ccw
  line L271 (299.8938, 92.225) -> (299.8938, 79.225)
  arc A265 (299.3938, 78.725) -> (299.8938, 79.225) centre (299.3938, 79.225) ccw
  line L272 (299.3938, 78.725) -> (286.3938, 78.725)
  arc A266 (159.6875, 3.025) -> (160.1875, 2.525) centre (160.1875, 3.025) ccw
  line L273 (159.6875, 3.025) -> (159.6875, 16.025)
  arc A267 (160.1875, 16.525) -> (159.6875, 16.025) centre (160.1875, 16.025) ccw
  line L274 (160.1875, 16.525) -> (173.1875, 16.525)
  arc A268 (173.6875, 16.025) -> (173.1875, 16.525) centre (173.1875, 16.025) ccw
  line L275 (173.6875, 16.025) -> (173.6875, 3.025)
  arc A269 (173.1875, 2.525) -> (173.6875, 3.025) centre (173.1875, 3.025) ccw
  line L276 (173.1875, 2.525) -> (160.1875, 2.525)
  arc A270 (359.7125, 79.225) -> (360.2125, 78.725) centre (360.2125, 79.225) ccw
  line L277 (359.7125, 79.225) -> (359.7125, 92.225)
  arc A271 (360.2125, 92.725) -> (359.7125, 92.225) centre (360.2125, 92.225) ccw
  line L278 (360.2125, 92.725) -> (373.2125, 92.725)
  arc A272 (373.7125, 92.225) -> (373.2125, 92.725) centre (373.2125, 92.225) ccw
  line L279 (373.7125, 92.225) -> (373.7125, 79.225)
  arc A273 (373.2125, 78.725) -> (373.7125, 79.225) centre (373.2125, 79.225) ccw
  line L280 (373.2125, 78.725) -> (360.2125, 78.725)
  arc A274 (282.725, 40.625) -> (283.225, 41.125) centre (282.725, 41.125) ccw
  line L281 (282.725, 40.625) -> (269.725, 40.625)
  arc A275 (269.225, 41.125) -> (269.725, 40.625) centre (269.725, 41.125) ccw
  line L282 (269.225, 41.125) -> (269.225, 54.125)
  arc A276 (269.725, 54.625) -> (269.225, 54.125) centre (269.725, 54.125) ccw
  line L283 (269.725, 54.625) -> (282.725, 54.625)
  arc A277 (283.225, 54.125) -> (282.725, 54.625) centre (282.725, 54.125) ccw
  line L284 (283.225, 54.125) -> (283.225, 41.125)
  arc A278 (83.4875, 3.025) -> (83.9875, 2.525) centre (83.9875, 3.025) ccw
  line L285 (83.4875, 3.025) -> (83.4875, 16.025)
  arc A279 (83.9875, 16.525) -> (83.4875, 16.025) centre (83.9875, 16.025) ccw
  line L286 (83.9875, 16.525) -> (96.9875, 16.525)
  arc A280 (97.4875, 16.025) -> (96.9875, 16.525) centre (96.9875, 16.025) ccw
  line L287 (97.4875, 16.025) -> (97.4875, 3.025)
  arc A281 (96.9875, 2.525) -> (97.4875, 3.025) centre (96.9875, 3.025) ccw
  line L288 (96.9875, 2.525) -> (83.9875, 2.525)
  arc A282 (64.4375, 3.025) -> (64.9375, 2.525) centre (64.9375, 3.025) ccw
  line L289 (64.4375, 3.025) -> (64.4375, 16.025)
  arc A283 (64.9375, 16.525) -> (64.4375, 16.025) centre (64.9375, 16.025) ccw
  line L290 (64.9375, 16.525) -> (77.9375, 16.525)
  arc A284 (78.4375, 16.025) -> (77.9375, 16.525) centre (77.9375, 16.025) ccw
  line L291 (78.4375, 16.025) -> (78.4375, 3.025)
  arc A285 (77.9375, 2.525) -> (78.4375, 3.025) centre (77.9375, 3.025) ccw
  line L292 (77.9375, 2.525) -> (64.9375, 2.525)
  arc A286 (340.6625, 79.225) -> (341.1625, 78.725) centre (341.1625, 79.225) ccw
  line L293 (340.6625, 79.225) -> (340.6625, 92.225)
  arc A287 (341.1625, 92.725) -> (340.6625, 92.225) centre (341.1625, 92.225) ccw
  line L294 (341.1625, 92.725) -> (354.1625, 92.725)
  arc A288 (354.6625, 92.225) -> (354.1625, 92.725) centre (354.1625, 92.225) ccw
  line L295 (354.6625, 92.225) -> (354.6625, 79.225)
  arc A289 (354.1625, 78.725) -> (354.6625, 79.225) centre (354.1625, 79.225) ccw
  line L296 (354.1625, 78.725) -> (341.1625, 78.725)
  arc A290 (140.6375, 3.025) -> (141.1375, 2.525) centre (141.1375, 3.025) ccw
  line L297 (140.6375, 3.025) -> (140.6375, 16.025)
  arc A291 (141.1375, 16.525) -> (140.6375, 16.025) centre (141.1375, 16.025) ccw
  line L298 (141.1375, 16.525) -> (154.1375, 16.525)
  arc A292 (154.6375, 16.025) -> (154.1375, 16.525) centre (154.1375, 16.025) ccw
  line L299 (154.6375, 16.025) -> (154.6375, 3.025)
  arc A293 (154.1375, 2.525) -> (154.6375, 3.025) centre (154.1375, 3.025) ccw
  line L300 (154.1375, 2.525) -> (141.1375, 2.525)
  arc A294 (178.7375, 3.025) -> (179.2375, 2.525) centre (179.2375, 3.025) ccw
  line L301 (178.7375, 3.025) -> (178.7375, 16.025)
  arc A295 (179.2375, 16.525) -> (178.7375, 16.025) centre (179.2375, 16.025) ccw
  line L302 (179.2375, 16.525) -> (192.2375, 16.525)
  arc A296 (192.7375, 16.025) -> (192.2375, 16.525) centre (192.2375, 16.025) ccw
  line L303 (192.7375, 16.025) -> (192.7375, 3.025)
  arc A297 (192.2375, 2.525) -> (192.7375, 3.025) centre (192.2375, 3.025) ccw
  line L304 (192.2375, 2.525) -> (179.2375, 2.525)
  arc A298 (197.7875, 3.025) -> (198.2875, 2.525) centre (198.2875, 3.025) ccw
  line L305 (197.7875, 3.025) -> (197.7875, 16.025)
  arc A299 (198.2875, 16.525) -> (197.7875, 16.025) centre (198.2875, 16.025) ccw
  line L306 (198.2875, 16.525) -> (211.2875, 16.525)
  arc A300 (211.7875, 16.025) -> (211.2875, 16.525) centre (211.2875, 16.025) ccw
  line L307 (211.7875, 16.025) -> (211.7875, 3.025)
  arc A301 (211.2875, 2.525) -> (211.7875, 3.025) centre (211.2875, 3.025) ccw
  line L308 (211.2875, 2.525) -> (198.2875, 2.525)
  arc A302 (116.0375, 2.525) -> (116.5375, 3.025) centre (116.0375, 3.025) ccw
  line L309 (116.0375, 2.525) -> (103.0375, 2.525)
  arc A303 (102.5375, 3.025) -> (103.0375, 2.525) centre (103.0375, 3.025) ccw
  line L310 (102.5375, 3.025) -> (102.5375, 16.025)
  arc A304 (103.0375, 16.525) -> (102.5375, 16.025) centre (103.0375, 16.025) ccw
  line L311 (103.0375, 16.525) -> (116.0375, 16.525)
  arc A305 (116.5375, 16.025) -> (116.0375, 16.525) centre (116.0375, 16.025) ccw
  line L312 (116.5375, 16.025) -> (116.5375, 3.025)
  arc A306 (45.3875, 3.025) -> (45.8875, 2.525) centre (45.8875, 3.025) ccw
  line L313 (45.3875, 3.025) -> (45.3875, 16.025)
  arc A307 (45.8875, 16.525) -> (45.3875, 16.025) centre (45.8875, 16.025) ccw
  line L314 (45.8875, 16.525) -> (58.8875, 16.525)
  arc A308 (59.3875, 16.025) -> (58.8875, 16.525) centre (58.8875, 16.025) ccw
  line L315 (59.3875, 16.025) -> (59.3875, 3.025)
  arc A309 (58.8875, 2.525) -> (59.3875, 3.025) centre (58.8875, 3.025) ccw
  line L316 (58.8875, 2.525) -> (45.8875, 2.525)
  arc A310 (216.8375, 3.025) -> (217.3375, 2.525) centre (217.3375, 3.025) ccw
  line L317 (216.8375, 3.025) -> (216.8375, 16.025)
  arc A311 (217.3375, 16.525) -> (216.8375, 16.025) centre (217.3375, 16.025) ccw
  line L318 (217.3375, 16.525) -> (230.3375, 16.525)
  arc A312 (230.8375, 16.025) -> (230.3375, 16.525) centre (230.3375, 16.025) ccw
  line L319 (230.8375, 16.025) -> (230.8375, 3.025)
  arc A313 (230.3375, 2.525) -> (230.8375, 3.025) centre (230.3375, 3.025) ccw
  line L320 (230.3375, 2.525) -> (217.3375, 2.525)
  arc A314 (61.2687, 78.725) -> (61.7687, 79.225) centre (61.2687, 79.225) ccw
  line L321 (61.2687, 78.725) -> (48.2687, 78.725)
  arc A315 (47.7688, 79.225) -> (48.2688, 78.725) centre (48.2688, 79.225) ccw
  line L322 (47.7688, 79.225) -> (47.7688, 92.225)
  arc A316 (48.2688, 92.725) -> (47.7687, 92.225) centre (48.2688, 92.225) ccw
  line L323 (48.2688, 92.725) -> (61.2688, 92.725)
  arc A317 (61.7688, 92.225) -> (61.2687, 92.725) centre (61.2687, 92.225) ccw
  line L324 (61.7688, 92.225) -> (61.7688, 79.225)
  line L325 (40.3875, 97.725) -> (40.3875, -2.475)
  line L326 (40.3875, -2.475) -> (475.8604, -2.475)
  line L327 (475.8604, -2.475) -> (475.8604, 97.725)
  line L328 (475.8604, 97.725) -> (40.3875, 97.725)
  line L329 (455.4341, 95.225) -> (42.8875, 95.225)
  line L330 (42.8875, 95.225) -> (42.8875, -0.6022)
  line L331 (44.5689, -2.475) -> (44.5689, 0.025)
  line L332 (42.8875, -0.6022) -> (373.0449, -0.4051)
  line L333 (380.0407, 6.5991) -> (380.029, 26.1497)
  arc A318 (387.2231, 33.1512) -> (380.029, 26.1497) centre (387.029, 26.1539) ccw
  line L334 (387.2231, 33.1512) -> (461.4345, 33.1955)
  arc A319 (461.4345, 33.1955) -> (468.4304, 40.1955) centre (461.4304, 40.1955) ccw
  line L335 (468.4304, 40.1955) -> (468.4304, 51.5909)
  arc A320 (468.4304, 51.5909) -> (465.4322, 57.3342) centre (461.4304, 51.5909) ccw
  arc A321 (462.4341, 63.0774) -> (465.4322, 57.3342) centre (469.4341, 63.0774) ccw
  line L336 (462.4341, 63.0774) -> (462.4341, 88.225)
  arc A322 (462.4341, 88.225) -> (455.4341, 95.225) centre (455.4341, 88.225) ccw
  arc A323 (373.0449, -0.4051) -> (380.0407, 6.5991) centre (373.0407, 6.5949) ccw
  dimension "d28" = 2.5
  dimension "d29" = 7
  dimension "d30" = 2.5
  constraint perpendicular L325 L329
  constraint perpendicular L326 L330
  constraint coincident L326 L331.start
  constraint perpendicular L326 L331
  constraint perpendicular L332 L333
  constraint tangent L333 A318
  constraint parallel L332 L334
  constraint tangent L334 A319
  constraint perpendicular L329 L335
  constraint tangent L335 A320
  constraint tangent A320 A321
  constraint parallel L212 L336
  constraint tangent L336 A322
  constraint equal A319 A320
  constraint equal A320 A321
  constraint equal A321 A322
  constraint equal A318 A319
  constraint tangent L333 A323
  constraint tangent L332 A323
  constraint equal A318 A323
  constraint tangent A319 L335
  constraint tangent A321 L336
  constraint tangent L329 A322
  measures "d28" distance of L331.start L331.end
  measures "d29" radius of A323
  measures "d30" distance of L328 L329
extrude "Extrude1'" add sketch "Sketch2" along normal blind 3 separate body contours L325 L326 L327 L328 makes body 2 in component "PCB fill Top"
extrude "Extrude1''" add 1 faces at (439.0883, -12.1078, -3) along direction (0, 0, -1) blind 3 separate body on bodies 2 makes body 3 in component "PCB fill Bottom"
sketch "Sketch3" plane through (0, 0, -6) normal (0, 0, -1) x (1, 0, 0)
  line L0 (462.4341, 88.225) -> (462.4341, 63.0774)
  arc A0 (462.4341, 63.0774) -> (465.4322, 57.3342) centre (469.4341, 63.0774) ccw
  arc A1 (468.4304, 51.5909) -> (465.4322, 57.3342) centre (461.4304, 51.5909) ccw
  line L1 (468.4304, 51.5909) -> (468.4304, 40.1955)
  arc A2 (461.4345, 33.1955) -> (468.4304, 40.1955) centre (461.4304, 40.1955) ccw
  line L2 (461.4345, 33.1955) -> (387.2231, 33.1512)
  arc A3 (387.2231, 33.1512) -> (380.029, 26.1497) centre (387.029, 26.1539) ccw
  line L3 (380.029, 26.1497) -> (380.0407, 6.5991)
  arc A4 (373.0449, -0.4051) -> (380.0407, 6.5991) centre (373.0407, 6.5949) ccw
  line L4 (373.0449, -0.4051) -> (42.8875, -0.6022)
  line L5 (42.8875, -0.6022) -> (42.8875, 95.225)
  line L6 (42.8875, 95.225) -> (455.4341, 95.225)
  arc A5 (462.4341, 88.225) -> (455.4341, 95.225) centre (455.4341, 88.225) ccw
  line L7 (475.8604, 97.725) -> (40.3875, 97.725)
  line L8 (40.3875, 97.725) -> (40.3875, -2.475)
  line L9 (40.3875, -2.475) -> (475.8604, -2.475)
  line L10 (475.8604, -2.475) -> (475.8604, 97.725)
  line L11 (475.8604, -2.475) -> (40.3875, -2.475)
  line L12 (40.3875, -2.475) -> (40.3875, 97.725)
  line L13 (40.3875, 97.725) -> (475.8604, 97.725)
  line L14 (475.8604, 97.725) -> (475.8604, -2.475)
  line L15 (383.7929, 34.7152, -6) -> (383.7929, 34.7152, 0)
  line L16 (383.7929, 34.7152) -> (459.7929, 34.7152)
  line L17 (459.7929, 34.7152) -> (459.8165, 93.6834)
  line L18 (383.7929, 34.7152) -> (383.7929, 95.225)
  line L19 (383.7929, 88.7152, -6) -> (383.7929, 88.7152, 0)
  line L20 (459.8145, 88.7152) -> (383.7929, 88.7152)
  point P0 (383.7929, 34.7152)
  point P1 (383.7929, 88.7152)
  dimension "d35" = 6
  dimension "d36" = 76
  constraint horizontal L11
  constraint vertical L12
  constraint horizontal L13
  constraint vertical L14
  constraint coincident L7.end L8.start
  constraint coincident L9.end L10.start
  constraint coincident P0 L16.start
  constraint coincident A5 L17.end
  constraint coincident L6 L18.end
  constraint perpendicular L6 L18
  constraint coincident P1 L20.end
  constraint coincident L18 P1
  constraint coincident L17 L20.start
  constraint perpendicular L18 L20
  measures "d35" distance of P0 L16.start
  measures "d36" distance of P0 L16.end
extrude "Extrude1'''" add sketch "Sketch3" along normal blind 3 separate body contours L0 A0 A1 L1 A2 L2 A3 L3 A4 L4 L5 L6 A5 L16 L17 L18 | L6 A5 L17 L18 L20 | L16 L17 L18 L20 | L7 L8 L9 L10 L11 L12 L13 L14 makes body 4 in component "Bottom plate"
sketch "Sketch4" plane through (0, 0, -9) normal (0, 0, -1) x (1, 0, 0)
  line L0 (475.8604, 97.725) -> (40.3875, 97.725)
  line L1 (40.3875, 97.725) -> (40.3875, -2.475)
  line L2 (40.3875, -2.475) -> (475.8604, -2.475)
  line L3 (475.8604, -2.475) -> (475.8604, 97.725)
  line L4 (475.8604, 47.625) -> (40.3875, 47.625)
  constraint midpoint L3 L4.start
  constraint midpoint L1 L4.end
extrude "Extrude1''''" add sketch "Sketch4" along normal blind 3 separate body contours L1 L2 L3 L4 makes body 5 in component "Top Standoff"
sketch "Sketch5" plane through (0, 0, -12) normal (0, 0, -1) x (1, 0, 0)
  line L0 (475.8604, 47.625) -> (40.3875, 47.625)
  line L1 (40.3875, 47.625) -> (40.3875, -2.475)
  line L2 (40.3875, -2.475) -> (475.8604, -2.475)
  line L3 (475.8604, -2.475) -> (475.8604, 47.625)
  line L4 (475.8604, 22.575) -> (40.3875, 22.575)
  constraint midpoint L3 L4.start
  constraint midpoint L1 L4.end
extrude "Extrude1'''''" add sketch "Sketch5" along normal blind 3 separate body contours L1 L2 L3 L4 makes body 6 in component "Bottom Standoff"
move_body "Move1" bodies 6 to x (1, 0, 0) y (0, 1, 0) z (0, 0, 1) at (0, 0, -33) in component "Bottom Standoff"
move_body "Move1'" bodies 5 to x (1, 0, 0) y (0, 1, 0) z (0, 0, 1) at (0, 0, 18) in component "Top Standoff"
move_body "Move2" bodies 6 to x (1, 0, 0) y (0, 1, 0) z (0, 0, 1) at (0, 0, 18) in component "Bottom Standoff"
move_body "Move1''" bodies 3 to x (1, 0, 0) y (0, 1, 0) z (0, 0, 1) at (0, 0, 5) in component "PCB fill Bottom"
move_body "Move1'''" bodies 4 to x (1, 0, 0) y (0, 1, 0) z (0, 0, 1) at (0, 0, 5) in component "Bottom plate"
move_body "Move2'" bodies 5 to x (1, 0, 0) y (0, 1, 0) z (0, 0, 1) at (0, 0, 5) in component "Top Standoff"
move_body "Move1''''" bodies 2 to x (1, 0, 0) y (0, 1, 0) z (0, 0, 1) at (0, 0, 5) in component "PCB fill Top"
move_body "Move1'''''" bodies 1 to x (1, 0, 0) y (0, 1, 0) z (0, 0, 1) at (0, 0, 5) in component "Plate"
move_body "Move2''" bodies 3 to x (1, 0, 0) y (0, 1, 0) z (0, 0, 1) at (0, 0, 5) in component "PCB fill Bottom"
move_body "Move2'''" bodies 4 to x (1, 0, 0) y (0, 1, 0) z (0, 0, 1) at (0, 0, 5) in component "Bottom plate"
move_body "Move2''''" bodies 2 to x (1, 0, 0) y (0, 1, 0) z (0, 0, 1) at (0, 0, 5) in component "PCB fill Top"
move_body "Move2'''''" bodies 1 to x (1, 0, 0) y (0, 1, 0) z (0, 0, 1) at (0, 0, 5) in component "Plate"
move_body "Move3" bodies 3 to x (1, 0, 0) y (0, 1, 0) z (0, 0, 1) at (0, 0, 5) in component "PCB fill Bottom"
move_body "Move3'" bodies 2 to x (1, 0, 0) y (0, 1, 0) z (0, 0, 1) at (0, 0, 5) in component "PCB fill Top"
move_body "Move3''" bodies 1 to x (1, 0, 0) y (0, 1, 0) z (0, 0, 1) at (0, 0, 5) in component "Plate"
move_body "Move4" bodies 2 to x (1, 0, 0) y (0, 1, 0) z (0, 0, 1) at (0, 0, 5) in component "PCB fill Top"
move_body "Move4'" bodies 1 to x (1, 0, 0) y (0, 1, 0) z (0, 0, 1) at (0, 0, 5) in component "Plate"